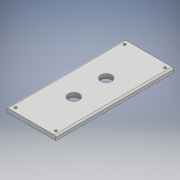
# Autodesk Inventor part: ICE CREAM COVER
Saved by Autodesk Inventor 2017 (Build 210142000, 142)
## iProperties
Created: 2019-09-14
Part Number: ICE CREAM COVER
Material: Generic
Document SubType Name: Modeling
Designer: Admin
Density: 1 g/cm^3
Appearance: Default
Mass: 38.3144 g
Surface Area: 177.371 cm^2
Volume: 38.3144 cm^3
Author: Admin
Autodesk Inventor part; units mm, degrees
ref_plane "YZ Plane" through (0, 0, 0) normal (1, 0, 0) x (0, 1, 0)
ref_plane "XZ Plane" through (0, 0, 0) normal (0, 1, 0) x (-1, 0, 0)
ref_plane "XY Plane" through (0, 0, 0) normal (0, 0, 1) x (1, 0, 0)
sketch "Sketch1" plane through (0, 0, 0) normal (0, 0, 1) x (1, 0, 0)
  line L0 (0, 0) -> (58, 0)
  line L1 (58, 0) -> (58, 138)
  line L2 (58, 138) -> (0, 138)
  line L3 (0, 138) -> (0, 0)
  dimension "d0" = 58
  dimension "d1" = 138
  constraints: 8 end point, 3 perpendicular, 1 horizontal
  measures "d0" distance of L0.start L0.end
  measures "d1" distance of L0.end L1.end
extrude "Extrusion1" add sketch "Sketch1" along normal blind 5
sketch "Sketch2" plane through (0, 0, 5) normal (0, 0, 1) x (1, 0, 0)
  circle A0 centre (53, 5) radius 1.5
  circle A1 centre (5.8194, 5) radius 1.5
  line L0 (58, 138) -> (0, 138) projected
  line L1 (0, 138) -> (0, 0) projected
  circle A2 centre (5.4959, 133) radius 1.5
  line L2 (58, 0) -> (58, 138) projected
  circle A3 centre (53, 133) radius 1.5
  dimension "d6" = 3
  dimension "d8" = 3
  dimension "d10" = 3
  dimension "d13" = 3
  constraints: 4 centre point
  measures "d6" diameter of A0
  measures "d8" diameter of A1
  measures "d10" diameter of A2
  measures "d13" diameter of A3
extrude "Extrusion2" cut sketch "Sketch2" against normal through all
fillet "Fillet1" radius 2 2 edges at (58, 69, 5) (0, 69, 5)
sketch "Sketch3" plane through (0, 0, 5) normal (0, 0, 1) x (1, 0, 0)
  line L0 (56, 138) -> (2, 138) projected
  circle A0 centre (29, 88) radius 6.5
  line L1 (0, 0) -> (58, 0) projected
  circle A1 centre (29, 50) radius 6.5
  dimension "d18" = 13
  dimension "d20" = 13
  constraints: 2 centre point
  measures "d18" diameter of A0
  measures "d20" diameter of A1
extrude "Extrusion3" cut sketch "Sketch3" against normal through all
body "Solid1"
